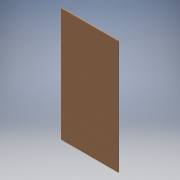
# Autodesk Inventor part: Türblatt
Saved by Autodesk Inventor 2017 (Build 210142000, 142)
## iProperties
Created: 2017-06-02
Part Number: Türblatt
Material: Holz (Kirsche)
Document SubType Name: Modeling
Designer: Fake
Density: 0.63 g/cm^3
Appearance: Kirsche - natur - schwacher Glanz
Author: Fake
Autodesk Inventor part; units mm, degrees
ref_plane "YZ Plane" through (0, 0, 0) normal (1, 0, 0) x (0, 1, 0)
ref_plane "XZ Plane" through (0, 0, 0) normal (0, 1, 0) x (-1, 0, 0)
ref_plane "XY Plane" through (0, 0, 0) normal (0, 0, 1) x (1, 0, 0)
sketch "Skizze1" plane through (0, 0, 0) normal (0, 1, 0) x (-1, 0, 0)
  line L0 (460, -980) -> (460, 905) projected
  line L1 (460, 905) -> (-460, 905) projected
  line L2 (-460, 905) -> (-460, -980) projected
  line L3 (480, -980) -> (-480, -980)
  line L4 (-480, -980) -> (-480, 925)
  line L5 (-480, 925) -> (480, 925)
  line L6 (480, 925) -> (480, -980)
  line L7 (0, -1361) -> (0, 1306) projected
  line L8 (672, 0) -> (-672, 0) projected
  dimension "d0" = 20
  dimension "d1" = 20
  dimension "d2" = 20
  constraints: 8 end point, 2 parallel, 1 horizontal, 1 perpendicular, 1 point on line
  measures "d0" distance between parallel lines of L0 L6
  measures "d1" distance between parallel lines of L1 L5
  measures "d2" distance between parallel lines of L4 L2
extrude "Extrusion1" add sketch "Skizze1" against normal blind 15
equation "\"d2\" = d0"
